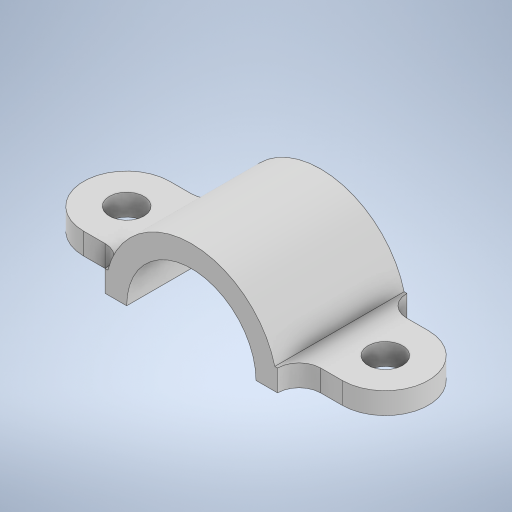
# Autodesk Inventor part: 4
Saved by Autodesk Inventor 2023 (Build 270158000, 158)
## iProperties
Created: 2023-10-10
Part Number: 4
Material: Všeobecné
Document SubType Name: Modeling
Designer: clu40164
Mass: 91.8818 g
Surface Area: 239.212 cm^2
Volume: 91.8818 cm^3
Density: 1 g/cm^3
Appearance: Výchozí
Author: clu40164
Autodesk Inventor part; units mm, degrees
ref_plane "YZ Plane" through (0, 0, 0) normal (1, 0, 0) x (0, 1, 0)
ref_plane "XZ Plane" through (0, 0, 0) normal (0, 1, 0) x (-1, 0, 0)
ref_plane "XY Plane" through (0, 0, 0) normal (0, 0, 1) x (1, 0, 0)
sketch "Náčrt2" plane through (0, 0, 0) normal (0, 0, 1) x (1, 0, 0)
  arc A0 (30, 0) -> (-30, 0) centre (0, 0) ccw
  arc A1 (40, 0) -> (-40, 0) centre (0, 0) ccw
  line L0 (-40, 0) -> (-30, 0)
  line L1 (30, 0) -> (40, 0)
  point P0 (-40, 0)
  dimension "d0" = 30
  dimension "d1" = 40
  dimension "d2" = 0
  dimension "d3" = 0
  dimension "d4" = 0
  dimension "d5" = 0
  dimension "d6" = 30
  dimension "d7" = 40
  constraints: 4 end point, 4 point on circle, 2 centre point, 2 coincident, 1 collinear, 1 horizontal
  measures "d0" radius of A0
  measures "d1" radius of A1
  measures "d2" distance between parallel lines of L0 L1
  measures "d3" distance from line of point (0, 0) L1
  measures "d4" distance from line of A0.start L1
  measures "d5" distance from line of A1.end L1
  measures "d6" distance of L1.start point (0, 0)
  measures "d7" distance of L0.start point (0, 0)
extrude "Vysunutí1" add sketch "Náčrt2" against normal blind 60
sketch "Náčrt3" plane through (30, 0, 0) normal (0, -1, 0) x (1, 0, 0)
  line L0 (10, 0) -> (-70, 0) projected
  line L1 (0, 0) -> (0, -60)
  line L2 (0, -60) -> (10, -60)
  line L3 (0, 0) -> (10, 0)
  line L4 (10, 0) -> (10, -60) projected
  line L5 (10, -60) -> (10, -60)
  line L6 (20, -50) -> (30, -50)
  line L7 (30, -10) -> (20, -10)
  line L8 (10, 0) -> (10, 0)
  arc A0 (30, -50) -> (30, -10) centre (30, -30) ccw
  circle A1 centre (30, -30) radius 8
  arc A2 (20, -50) -> (10, -60) centre (20, -60) ccw
  arc A3 (10, 0) -> (20, -10) centre (20, 0) ccw
  line L9 (-30, 0) -> (-30, -60)
  line L10 (-60, 0) -> (-60, -60)
  line L11 (-60, -60) -> (-70, -60)
  line L12 (-60, 0) -> (-70, 0)
  line L13 (-70, 0) -> (-70, -60)
  line L14 (-70, -60) -> (-70, -60)
  line L15 (-80, -50) -> (-90, -50)
  line L16 (-90, -10) -> (-80, -10)
  line L17 (-70, 0) -> (-70, 0)
  arc A4 (-90, -10) -> (-90, -50) centre (-90, -30) ccw
  circle A5 centre (-90, -30) radius 8
  arc A6 (-70, -60) -> (-80, -50) centre (-80, -60) ccw
  arc A7 (-80, -10) -> (-70, 0) centre (-80, 0) ccw
  point P0 (10, -50)
  point P1 (10, -10)
  point P2 (-70, -50)
  point P3 (-70, -10)
  dimension "d10" = 10
  dimension "d12" = 16
  dimension "d13" = 10
  dimension "d16" = 20
  dimension "d17" = 30
  constraints: 32 end point, 16 symmetric about line, 13 point on line, 12 point on circle, 8 centre point, 6 tangent, 3 vertical, 2 coincident, 2 horizontal, 1 equal radius, 1 parallel, 1 perpendicular, 4 other
  measures "d10" distance of point (10, -50) L2.end
  measures "d12" diameter of A1
  measures "d13" radius of A2
  measures "d16" distance of L7.start A0.centre
  measures "d17" distance from line of L1 A0.centre
extrude "Vysunutí2" add sketch "Náčrt3" against normal blind 10
